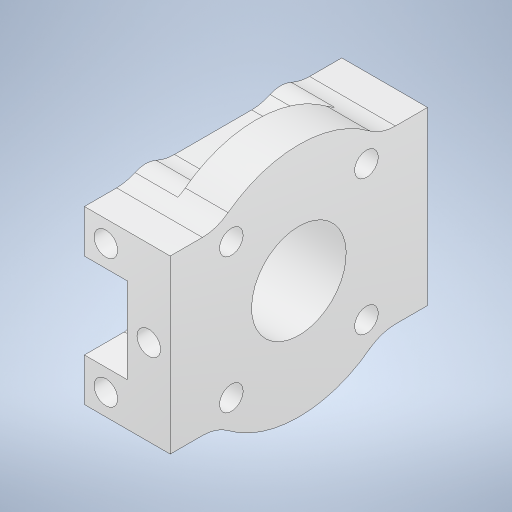
# Autodesk Inventor part: Bracket
Saved by Autodesk Inventor 2023.2 (Build 272271000, 271)
## iProperties
Created: 2024-01-11
Part Number: Bracket
Material: Aluminum 6061
Document SubType Name: Modeling
Designer: Nathan Cai
Mass: 30.4757 g
Surface Area: 53.4519 cm^2
Volume: 11.2873 cm^3
Density: 2.7 g/cm^3
Appearance: Aluminum - Flat
Author: Nathan Cai
Autodesk Inventor part; units mm, degrees
ref_plane "YZ Plane" through (0, 0, 0) normal (1, 0, 0) x (0, 1, 0)
ref_plane "XZ Plane" through (0, 0, 0) normal (0, 1, 0) x (-1, 0, 0)
ref_plane "XY Plane" through (0, 0, 0) normal (0, 0, 1) x (1, 0, 0)
sketch "Sketch1" plane through (0, 0, 0) normal (1, 0, 0) x (0, 1, 0)
  line L0 (-12.7, 19.05) -> (12.7, 19.05)
  line L1 (12.7, 19.05) -> (12.7, -19.05)
  line L2 (12.7, -19.05) -> (-12.7, -19.05)
  line L3 (-12.7, -19.05) -> (-12.7, 19.05)
  line L4 (-12.7, 19.05) -> (12.7, -19.05) construction
  line L5 (12.7, 19.05) -> (-12.7, -19.05) construction
  line L6 (-10, 10) -> (10, 10) construction
  line L7 (10, 10) -> (10, -10) construction
  line L8 (10, -10) -> (-10, -10) construction
  line L9 (-10, -10) -> (-10, 10) construction
  line L10 (-10, 10) -> (10, -10) construction
  line L11 (10, 10) -> (-10, -10) construction
  circle A0 centre (10, 10) radius 1.7526
  circle A1 centre (-10, 10) radius 1.7526
  circle A2 centre (-10, -10) radius 1.7526
  circle A3 centre (10, -10) radius 1.7526
  circle A4 centre (0, 0) radius 17.4625
  circle A5 centre (0, 0) radius 7
  point P0 (-12.7, 11.9854)
  point P1 (-12.7, -11.9854)
  point P2 (12.7, -11.9854)
  point P3 (12.7, 11.9854)
  dimension "d0" = 25.4
  dimension "d1" = 38.1
  dimension "d2" = 20
  dimension "d3" = 20
  dimension "d4" = 3.5052
  dimension "d7" = 360
  dimension "d9" = 34.925
  dimension "d10" = 14
  constraints: 24 end point, 6 centre point, 5 coincident, 4 midpoint, 4 parallel, 2 horizontal, 2 perpendicular, 11 other
  measures "d0" distance of L1.end L2.end
  measures "d1" distance of L0.end L1.end
  measures "d2" distance of L7.end L8.end
  measures "d3" distance of L6.end L7.end
  measures "d4" diameter of A0
  measures "d9" diameter of A4
  measures "d10" diameter of A5
extrude "Extrusion1" add sketch "Sketch1" along normal blind 6.35
fillet "Fillet1" radius 6.35 4 edges at (3.175, 12.7, 11.9854) (3.175, 12.7, -11.9854) (3.175, -12.7, -11.9854) (3.175, -12.7, 11.9854)
sketch "Sketch3" plane through (0, 0, 0) normal (-1, 0, 0) x (0, 0, 1)
  circle A0 centre (-10, 10) radius 1.7526 projected
  circle A1 centre (-10, 10) radius 3.6642
  arc A2 (-14.2875, 12.7) -> (-10.4775, 13.97) centre (-14.2875, 19.05) ccw projected
  circle A3 centre (0, 0) radius 12.3895
  circle A4 centre (-10, -10) radius 3.6642
  circle A5 centre (10, -10) radius 3.6642
  circle A6 centre (10, 10) radius 3.6642
  line L0 (-19.05, 12.7) -> (-14.2875, 12.7) projected
  line L1 (19.05, 12.7) -> (19.05, -12.7) projected
  line L2 (-19.05, 12.7) -> (19.05, 12.7)
  line L3 (19.05, 12.7) -> (19.05, 6.3358)
  line L4 (19.05, 6.3358) -> (-19.05, 6.3358)
  line L5 (-19.05, 6.3358) -> (-19.05, 12.7)
  line L6 (-19.05, -12.7) -> (-19.05, 12.7) projected
  line L7 (19.05, -12.7) -> (-19.05, -12.7)
  line L8 (-19.05, -12.7) -> (-19.05, -6.3358)
  line L9 (-19.05, -6.3358) -> (19.05, -6.3358)
  line L10 (19.05, -6.3358) -> (19.05, -12.7)
  arc A7 (-10.4775, -13.97) -> (-14.2875, -12.7) centre (-14.2875, -19.05) ccw projected
  arc A8 (-10.4775, -13.97) -> (10.4775, -13.97) centre (0, 0) ccw projected
  arc A9 (14.2875, -12.7) -> (10.4775, -13.97) centre (14.2875, -19.05) ccw projected
  line L11 (19.05, -12.7) -> (14.2875, -12.7) projected
  line L12 (19.05, 12.7) -> (19.05, -12.7) projected
  line L13 (14.2875, 12.7) -> (19.05, 12.7) projected
  arc A10 (10.4775, 13.97) -> (14.2875, 12.7) centre (14.2875, 19.05) ccw projected
  arc A11 (10.4775, 13.97) -> (-10.4775, 13.97) centre (0, 0) ccw projected
  arc A12 (-14.2875, 12.7) -> (-10.4775, 13.97) centre (-14.2875, 19.05) ccw projected
  line L14 (-19.05, 12.7) -> (-14.2875, 12.7) projected
  line L15 (-19.05, -12.7) -> (-19.05, 12.7) projected
  line L16 (-14.2875, -12.7) -> (-19.05, -12.7) projected
  circle A13 centre (10, 10) radius 1.7526 projected
  circle A14 centre (10, -10) radius 1.7526 projected
  circle A15 centre (-10, -10) radius 1.7526 projected
  circle A16 centre (-10, 10) radius 1.7526 projected
  circle A17 centre (0, 0) radius 7 projected
  point P0 (-7.5228, 12.7)
  point P1 (-12.4772, 12.7)
  point P2 (-14.2875, 12.7)
  point P3 (-10.647, 6.3358)
  point P4 (-10.647, -6.3358)
  point P5 (-12.4772, -12.7)
  point P6 (-7.5228, -12.7)
  point P7 (7.5228, -12.7)
  point P8 (12.4772, -12.7)
  point P9 (10.647, -6.3358)
  point P10 (10.647, 6.3358)
  point P11 (12.4772, 12.7)
  point P12 (7.5228, 12.7)
  dimension "d22" = 360
  constraints: 16 end point, 5 centre point, 4 parallel, 4 tangent, 2 coincident, 2 horizontal, 2 perpendicular, 2 point on line, 9 other
extrude "Extrusion3" add sketch "Sketch3" along normal blind 6.35 contours A3 A1 L2 | A3 A1 | A3 A6 L4 A17 A1 | A1 L2 A6 A3 | A3 L4 L5 L0 L2 A1 | A1 L4 A3 | L2 A1 | A6 L2 A3 | A3 A6 | L4 A17 L9 A3 | A6 L2 | A6 A3 L4 | L4 A3 L9 A17 | L9 A4 A3 | A3 A4 L7 L6 L9 | L2 L1 L4 A3 A6 | A17 L9 A5 A3 A4 | A4 A3 | A3 A4 L7 | L7 A4 | L9 L1 L7 A5 A3 | A3 A5 L9 | A5 A3 | A3 A5 L7 A4 | A5 L7 A3 | L7 A5
fillet "Fillet2" radius 6.35 8 edges at (-3.175, -12.7, -12.4772) (-3.175, -12.7, 12.4772) (-3.175, 12.7, 12.4772) (-3.175, 12.7, -12.4772) (-3.175, -12.7, -7.5228) (-3.175, -12.7, 7.5228) (-3.175, 12.7, 7.5228) (-3.175, 12.7, -7.5228)
fillet "Fillet3" radius 1.5875 4 edges at (-3.175, -6.3358, 10.647) (-3.175, 6.3358, 10.647) (-3.175, -6.3358, -10.647) (-3.175, 6.3358, -10.647)
chamfer "Chamfer3" distance 1.5875 angle 45 4 edges at (-6.35, 10, -11.7526) (-6.35, 10, 8.2474) (-6.35, -10, -11.7526) (-6.35, -10, 8.2474)
sketch "Sketch4" plane through (6.35, -12.7, -19.05) normal (0, 0, -1) x (-1, 0, 0)
  line L0 (12.7, 25.4) -> (12.7, 19.0358) projected
  line L1 (12.5475, 22.225) -> (0, 22.225) construction
  line L2 (0, 0) -> (0, 25.4) projected
  line L3 (6.35, 12.7) -> (0, 12.7) construction
  line L4 (6.35, 19.0358) -> (12.7, 19.0358) projected
  line L5 (9.525, 19.0358) -> (9.525, 25.4) construction
  line L6 (12.7, 25.4) -> (0, 25.4) projected
  circle A0 centre (3.175, 12.7) radius 1.75
  line L7 (12.5475, 3.175) -> (0, 3.175) construction
  line L8 (9.525, 6.3642) -> (9.525, 0) construction
  circle A1 centre (9.525, 22.225) radius 1.75
  circle A2 centre (9.525, 3.175) radius 1.75
  dimension "d37" = 3.5
  dimension "d44" = 9.525
  dimension "d46" = 3.5
  constraints: 10 end point, 5 symmetric about line, 4 point on line, 3 centre point, 3 midpoint, 1 horizontal, 1 vertical, 1 other
  measures "d37" diameter of A0
  measures "d44" distance between parallel lines of L1 L3
  measures "d46" diameter of A1
extrude "Extrusion4" cut sketch "Sketch4" against normal blind 6
chamfer "Chamfer4" distance 1.75 angle 45 3 edges at (4.925, 0, -13.05) (-1.425, 9.525, -13.05) (-1.425, -9.525, -13.05)
mirror "Mirror1" about plane through (0, 0, 0) normal (0, 0, 1) of "Extrusion4", "Chamfer4"
body "Solid1"
